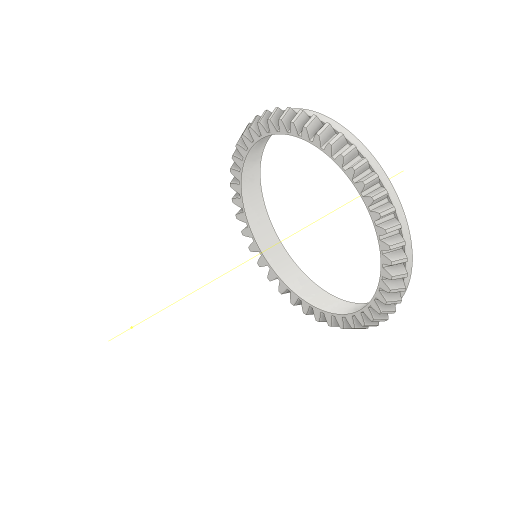
# Autodesk Inventor part: Bevel Gear1
Saved by Autodesk Inventor 2023 (Build 270158000, 158)
## iProperties
CustomPartVersion: 1
Created: 2023-05-08
Part Number: Bevel Gear1
Material: Steel, Mild
Document SubType Name: Modeling
Designer: Juyoung Han
Categories: <?xml version="1.0" encoding="UTF-16"?> <MemberInstance><Categories><FamilyTemplate><FamilyTemplateParameter ValueType="xs:double" Id="1" ObjectReferenceKey="da_z" ObjectType="kUserParameterObject"/><FamilyTemplateParameter ValueType="xs:double" Id="2" ObjectReferenceKey="da_b" ObjectType="kUserParameterObject"/><FamilyTemplateParameter ValueType="xs:double" Id="3" ObjectReferenceKey="da_beta" ObjectType="kUserParameterObject"/><FamilyTemplateParameter ValueType="xs:double" Id="4" ObjectReferenceKey="da_dae" ObjectType="kUserParameterObject"/><FamilyTemplateParameter ValueType="xs:double" Id="5" ObjectReferenceKey="da_ve" ObjectType="kUserParameterObject"/><FamilyTemplateParameter ValueType="xs:double" Id="6" ObjectReferenceKey="da_omega" ObjectType="kUserParameterObject"/><FamilyTemplateParameter ValueType="xs:string" Id="7" ObjectReferenceKey="EAIAABAAAAAAHwAAAAAAAIAAAAAAAAAA" ObjectType="83914240" SubObjectId="SurfaceGeometry"/></FamilyTemplate><ParamToTemplateMap><ParamToTemplate CategoryParameter="//CategoryParameter[@InternalName='046C89C9-8512-4d59-83FE-43B91F4F132A']" TemplateParameter="1"/><ParamToTemplate CategoryParameter="//CategoryParameter[@InternalName='2552DF32-E462-4b46-AEBF-C6C7768E72AC']" TemplateParameter="2"/><ParamToTemplate CategoryParameter="//CategoryParameter[@InternalName='C9EE641D-15FC-4fae-A226-E94C4372FDD7']" TemplateParameter="3"/><ParamToTemplate><ParamToTemplate CategoryParameter="//CategoryParameter[@InternalName='00B6519A-459B-49c7-AD84-2E56D39A5744']" ConstantValue="0.000000"/></ParamToTemplate><ParamToTemplate><ParamToTemplate CategoryParameter="//CategoryParameter[@InternalName='04B31F0E-C7A6-4894-AA32-9629BEFACF47']" ConstantValue="1.000000"/></ParamToTemplate><ParamToTemplate><ParamToTemplate CategoryParameter="//CategoryParameter[@InternalName='43CBEC2E-7847-49e7-A936-2F7889FCB2D9']" ConstantValue="0.200000"/></ParamToTemplate><ParamToTemplate><ParamToTemplate CategoryParameter="//CategoryParameter[@InternalName='B1EFC894-105D-4ebd-86BF-FA20ED196853']" ConstantValue="0.300000"/></ParamToTemplate><ParamToTemplate><ParamToTemplate CategoryParameter="//CategoryParameter[@InternalName='51175063-3D10-4879-93E8-6246FE8B403D']" ConstantValue="2060000000.000000"/></ParamToTemplate><ParamToTemplate><ParamToTemplate CategoryParameter="//CategoryParameter[@InternalName='A3A52E27-4454-46a9-B0BD-C932399B70AF']" ConstantValue="0.300000"/></ParamToTemplate><ParamToTemplate CategoryParameter="//CategoryParameter[@InternalName='2A200944-5A8C-41ca-B96E-8520D2E510F1']" TemplateParameter="4"/><ParamToTemplate><ParamToTemplate CategoryParameter="//CategoryParameter[@InternalName='1A637F62-92C8-44bc-B81F-10802510B579']" ConstantValue="11.345646"/></ParamToTemplate><ParamToTemplate CategoryParameter="//CategoryParameter[@InternalName='B52DD4BE-6863-48fb-BF58-89EF6F9EC65C']" TemplateParameter="5"/><ParamToTemplate><ParamToTemplate CategoryParameter="//CategoryParameter[@InternalName='3956BFF2-84D2-457d-93C2-9B0613DEBA67']" ConstantValue="12.541217"/></ParamToTemplate><ParamToTemplate CategoryParameter="//CategoryParameter[@InternalName='739CFA02-461B-4bf8-8049-181FCAD8B28F']" TemplateParameter="6"/><ParamToTemplate><ParamToTemplate CategoryParameter="//CategoryParameter[@InternalName='A27E999F-E2CE-4481-8A2A-EBF499C4C3C5']" ConstantValue="0.000000"/></ParamToTemplate><ParamToTemplate><ParamToTemplate CategoryParameter="//CategoryParameter[@InternalName='9E1B4470-B2D3-4ff1-B813-535BB4CDF51A']" ConstantValue="3520000.000000"/></ParamToTemplate><ParamToTemplate><ParamToTemplate CategoryParameter="//CategoryParameter[@InternalName='F8452263-BFF6-458c-9FB1-07C4B99E95CD']" ConstantValue="11400000.000000"/></ParamToTemplate><ParamToTemplate><ParamToTemplate CategoryParameter="//CategoryParameter[@InternalName='3E3BB259-FD49-497f-8171-6EBC954A3479']" ConstantValue="2.000000"/></ParamToTemplate><ParamToTemplate CategoryParameter="//CategoryParameter[@InternalName='27C3BAF2-7550-4e4b-AE2C-0DB134B7D9B7']" TemplateParameter="7"/></ParamToTemplateMap><Category DisplayName="Gear" InternalName="DC85795E-93AB-48d5-8EEE-5A27447B64BD" Mnemonic="Gear"><CategoryParameter DisplayName="z" InternalName="046C89C9-8512-4d59-83FE-43B91F4F132A" Mnemonic="z"/><CategoryParameter DisplayName="b" InternalName="2552DF32-E462-4b46-AEBF-C6C7768E72AC" Mnemonic="b"/><CategoryParameter DisplayName="||b|" InternalName="C9EE641D-15FC-4fae-A226-E94C4372FDD7" Mnemonic="beta"/><CategoryParameter DisplayName="x" InternalName="00B6519A-459B-49c7-AD84-2E56D39A5744" Mnemonic="x"/><CategoryParameter DisplayName="a*" InternalName="04B31F0E-C7A6-4894-AA32-9629BEFACF47" Mnemonic="a"/><CategoryParameter DisplayName="c*" InternalName="43CBEC2E-7847-49e7-A936-2F7889FCB2D9" Mnemonic="c"/><CategoryParameter DisplayName="r|.f|*" InternalName="B1EFC894-105D-4ebd-86BF-FA20ED196853" Mnemonic="rf"/><CategoryParameter DisplayName="E" InternalName="51175063-3D10-4879-93E8-6246FE8B403D" Mnemonic="E"/><CategoryParameter DisplayName="||m|" InternalName="A3A52E27-4454-46a9-B0BD-C932399B70AF" Mnemonic="mi"/><Category DisplayName="BevelGear" InternalName="0C98F69A-0C2B-4791-B2FE-7691BB227E77" Mnemonic="BevelGear"><CategoryParameter DisplayName="d|.ae|" InternalName="2A200944-5A8C-41ca-B96E-8520D2E510F1" Mnemonic="dae"/><CategoryParameter DisplayName="d|.ai|" InternalName="1A637F62-92C8-44bc-B81F-10802510B579" Mnemonic="dai"/><CategoryParameter DisplayName="A|.e|" InternalName="B52DD4BE-6863-48fb-BF58-89EF6F9EC65C" Mnemonic="ve"/><CategoryParameter DisplayName="A|.i|" InternalName="3956BFF2-84D2-457d-93C2-9B0613DEBA67" Mnemonic="vi"/><CategoryParameter DisplayName="||S|" InternalName="739CFA02-461B-4bf8-8049-181FCAD8B28F" Mnemonic="omega"/><CategoryParameter DisplayName="x|.t|" InternalName="A27E999F-E2CE-4481-8A2A-EBF499C4C3C5" Mnemonic="xt"/><CategoryParameter DisplayName="||s||.Flim|" InternalName="9E1B4470-B2D3-4ff1-B813-535BB4CDF51A" Mnemonic="sFlim"/><CategoryParameter DisplayName="||s||.Hlim|" InternalName="F8452263-BFF6-458c-9FB1-07C4B99E95CD" Mnemonic="sHlim"/><CategoryParameter DisplayName="type" InternalName="3E3BB259-FD49-497f-8171-6EBC954A3479" Mnemonic="type"/><CategoryParameter DisplayName="PitchDiameter" InternalName="27C3BAF2-7550-4e4b-AE2C-0DB134B7D9B7" Mnemonic="IDS_PITCHDIAM"/></Category></Category></Categories></MemberInstance>
Mass: 523.27 g
Surface Area: 330.412 cm^2
Volume: 66.6586 cm^3
Density: 7.85 g/cm^3
Appearance: Steel
Author: Juyoung Han
Autodesk Inventor part; units mm, degrees
ref_plane "Mesh Plane2" through (0, 0, 0) normal (0.9969173, 0.0784591, 0) x (0, 0, 1)
sketch "Teeth Body Sketch" plane through (0, 0, 0) normal (1, 0, 0) x (0, 1, 0)
  line L0 (0, 0) -> (66.1399, -164.8988) construction
  line L1 (66.1399, -164.8988) -> (73.2167, -161.8642)
  line L2 (73.2167, -161.8642) -> (0, 0) construction
  line L3 (70, -163.2436) -> (0, 0) construction
  line L4 (51.2451, -127.7634) -> (56.7282, -125.4122)
  line L5 (66.1399, -164.8988) -> (51.2451, -127.7634)
  line L6 (73.2167, -161.8642) -> (56.7282, -125.4122)
  line L7 (0, -189.5529) -> (0, 31.5922) projected
  line L8 (0, -163.2436) -> (73.2167, -163.2436) construction
  dimension "d0" = 140
  dimension "d1" = 132.2798
  dimension "d2" = 146.4335
  dimension "d3" = 40
  dimension "d4" = 161.8642
  constraints: 16 end point, 4 point on line, 3 perpendicular, 2 collinear, 1 horizontal alignment, 1 vertical alignment
  measures "d0" diameter of L3.start L7
  measures "d1" diameter of L0.end L7
  measures "d2" diameter of L1.end L7
  measures "d3" distance between parallel lines of L1 L4
  measures "d4" vertical distance of L1.end L0.start
revolve "Teeth Body" add sketch "Teeth Body Sketch" angle 360 about axis through (0, 0, 0) along (0, 0, 1)
ref_plane "Tooth Plane" through (0, 70, -163.2436) normal (0, -0.3941023, 0.9190666) x (1, 0, 0)
sketch "Start Sketch" plane through (0, 70, -163.2436) normal (0, -0.3941023, 0.9190666) x (1, 0, 0)
  line L0 (0, -93.2145) -> (0, 22.3576) projected
  arc A0 (-1.2885, -5.124) -> (-5.8753, 5.5992) centre (-28.0588, -10.2322) ccw
  arc A1 (5.8753, 5.5992) -> (1.2885, -5.124) centre (28.0588, -10.2322) ccw
  line L1 (-1.2885, -5.124) -> (1.2885, -5.124)
  arc A2 (5.8753, 5.5992) -> (-5.8753, 5.5992) centre (0, -76.1642) ccw
  dimension "d7" = 27.2533
  dimension "d8" = 28.0588
  dimension "d9" = 65.932
  dimension "d57" = 81.9742
  dimension "d58" = 71.0402
  constraints: 6 point on circle, 3 centre point, 3 symmetric about line, 2 end point, 1 coincident, 1 perpendicular, 1 other
  measures "d7" radius of A0
  measures "d8" horizontal distance of point (0, -76.164) A0.centre
  measures "d9" vertical distance of point (0, -76.164) A0.centre
  measures "d57" radius of A2
  measures "d58" distance from line of A2.centre L1
sketch "End Sketch" plane through (0, 54.0842, -126.1271) normal (0, -0.3941023, 0.9190666) x (1, 0, 0)
  line L0 (0, -71.2267) -> (0, 17.0838) projected
  arc A0 (-0.9956, -3.959) -> (-4.5394, 4.3261) centre (-21.6791, -7.9057) ccw
  arc A1 (4.5394, 4.3261) -> (0.9956, -3.959) centre (21.6791, -7.9057) ccw
  line L1 (-0.9956, -3.959) -> (0.9956, -3.959)
  arc A2 (4.5394, 4.3261) -> (-4.5394, 4.3261) centre (0, -58.8469) ccw
  dimension "d12" = 21.0567
  dimension "d15" = 21.6791
  dimension "d16" = 50.9411
  dimension "d59" = 63.3358
  dimension "d60" = 54.8879
  constraints: 6 point on circle, 3 centre point, 3 symmetric about line, 2 end point, 1 coincident, 1 other
  measures "d12" radius of A0
  measures "d15" horizontal distance of A0.centre point (0, -58.847)
  measures "d16" vertical distance of A0.centre point (0, -58.847)
  measures "d59" radius of A2
  measures "d60" distance from line of A2.centre L1
loft "Loft" cut profiles "Start Sketch", "End Sketch"
pattern_circular "Circular Pattern" count 40 over 360 about axis through (0, 0, 0) along (0, 0, 1) of "Loft"
ref_plane "End Plane" through (0, 54.0842, -126.1271) normal (0, -0.3941023, 0.9190666) x (1, 0, 0)
sketch3d "3D Sketch Right"
ref_plane "End Plane Right" through (-12.8268, 52.5411, -126.1271) normal (0.0934666, -0.3828585, 0.9190666) x (0.9714698, 0.2371632, 0)
sketch "End Sketch Right" plane through (-12.8268, 52.5411, -126.1271) normal (0.0934666, -0.3828585, 0.9190666) x (0.9714698, 0.2371632, 0)
  arc A0 (-0.9956, -3.959) -> (-4.5394, 4.3261) centre (-21.6791, -7.9057) ccw
  line L0 (0, -84.3011) -> (0, 29.9223) projected
  arc A1 (4.5394, 4.3261) -> (0.9956, -3.959) centre (21.6791, -7.9057) ccw
  line L1 (-0.9956, -3.959) -> (0.9956, -3.959)
  arc A2 (4.5394, 4.3261) -> (-4.5394, 4.3261) centre (0, -58.8469) ccw
  dimension "d70" = 21.6791
  dimension "d71" = 50.9411
  dimension "d72" = 21.0567
  dimension "d73" = 54.8879
  dimension "d74" = 63.3358
  constraints: 6 point on circle, 3 centre point, 3 symmetric about line, 2 end point, 1 coincident, 1 perpendicular, 1 other
  measures "d70" horizontal distance of A2.centre A0.centre
  measures "d71" vertical distance of point (0, -58.847) A0.centre
  measures "d72" radius of A0
  measures "d73" distance from line of point (0, -58.847) L1
  measures "d74" radius of A2
feature "Loft Right" [suppressed]
pattern_circular "Circular Pattern Right" [suppressed]
sketch3d "3D Sketch Left"
ref_plane "End Plane Left" through (12.7774, 52.5411, -126.11) normal (-0.0931208, -0.382915, 0.9190782) x (0.9716797, -0.236302, 0)
sketch "End Sketch Left" plane through (12.7774, 52.5411, -126.11) normal (-0.0931208, -0.382915, 0.9190782) x (0.9716797, -0.236302, 0)
  line L0 (0, -153.675) -> (0, 58.45) projected
  arc A0 (-0.9956, -3.9549) -> (-4.5394, 4.3301) centre (-21.6791, -7.9017) ccw
  arc A1 (4.5394, 4.3301) -> (0.9956, -3.9549) centre (21.6791, -7.9017) ccw
  line L1 (-0.9956, -3.9549) -> (0.9956, -3.9549)
  ellipse E0 centre (0, -49.4218) end of major axis (56.7282, -49.4218) minor radius 52.1377 projected
  arc A2 (4.5394, 4.3301) -> (-4.5394, 4.3301) centre (0, -58.8428) ccw
  dimension "d56" = 52.1377
  dimension "d30" = 21.0567
  dimension "d31" = 21.6791
  dimension "d32" = 50.9411
  dimension "d61" = 63.3358
  dimension "d62" = 54.8879
  constraints: 6 point on circle, 3 centre point, 3 symmetric about line, 2 end point, 1 coincident, 2 other
  measures "d30" radius of A0
  measures "d31" horizontal distance of point (0, -58.843) A0.centre
  measures "d32" vertical distance of A0.centre point (0, -58.843)
  measures "d61" radius of A2
  measures "d62" distance from line of point (0, -58.843) L1
feature "Loft Left" [suppressed]
pattern_circular "Circular Pattern Left" [suppressed]
sketch "Body Sketch" plane through (0, 0, 0) normal (1, 0, 0) x (0, 1, 0)
  line L0 (0, -165.3418) -> (0, -113.6747) projected
  line L1 (66.1399, -164.8988) -> (51.2451, -127.7634) projected
  line L2 (51.2451, -127.7634) -> (0, -127.7634)
  line L3 (66.1399, -164.8988) -> (0, -164.8988)
  constraints: 4 end point, 2 perpendicular, 2 point on line
revolve "Fix Body" add sketch "Body Sketch" angle 360 about axis through (0, 0, 0) along (0, 0, 1)
sketch "Sketch6" plane through (0, 0, 0) normal (1, 0, 0) x (0, 1, 0)
  line L0 (70, -163.2436) -> (0, 0) projected
  line L1 (0, -187.4923) -> (0, 31.2487) projected
surface revolve "Pitch Diameter" sketch "Sketch6" angle 360 about axis through (0, 0, 0) along (0, 0, 1) shown no curves L0
sketch "Sketch8" plane through (0, 0, -127.7634) normal (0, 0, 1) x (0.9969173, 0.0784591, 0)
  circle A0 centre (0, 0) radius 78.8545
  constraints: 1 centre point, 1 coincident
extrude "Extrusion1" cut sketch "Sketch8" along normal blind 10 and the other way blind 25
sketch "Sketch9" plane through (0, 0, -164.8988) normal (0, 0, -1) x (-0.9969173, 0.0784591, 0)
  circle A0 centre (0, 0) radius 68.2
  dimension "d98" = 136.4
  constraints: 1 centre point, 1 coincident
  measures "d98" diameter of A0
extrude "Extrusion2" add sketch "Sketch9" along normal blind 6
sketch "Sketch10" plane through (0, 0, -170.8988) normal (0, 0, -1) x (-1, 0, 0)
  circle A0 centre (0, 0) radius 65.8
  dimension "d101" = 131.6
  constraints: 1 centre point, 1 coincident
  measures "d101" diameter of A0
extrude "Extrusion3" cut sketch "Sketch10" against normal blind 2
sketch "Sketch11" plane through (0, 0, -168.8988) normal (0, 0, -1) x (-1, 0, 0)
  circle A0 centre (0, 0) radius 59.5
  dimension "d104" = 119
  constraints: 1 centre point, 1 coincident
  measures "d104" diameter of A0
extrude "Extrusion4" cut sketch "Sketch11" against normal through all
equation "\"d0\" = da_de"
equation "\"d1\" = da_dfe"
equation "\"d2\" = da_dae"
equation "\"d3\" = da_b"
equation "\"d4\" = da_ve"
equation "\"d7\" = fd_rr"
equation "\"d8\" = fd_x"
equation "\"d9\" = fd_y"
equation "\"d57\" = 0.5 * fd_dva + 0.3 * da_he"
equation "\"d58\" = 0.5 * fd_dva - 1.12 * da_he"
equation "\"da_teethtype\" = 0"
equation "\"da_b\" = 40"
equation "\"da_de\" = 140"
equation "\"da_dae\" = 146.43347"
equation "\"da_dfe\" = 132.27984"
equation "\"da_le\" = 177.61886"
equation "\"da_omega\" = 30deg"
equation "\"da_beta\" = 0"
equation "\"da_delta\" = 23.209998deg"
equation "\"da_alpha\" = 20deg"
equation "\"da_he\" = 7.7"
equation "\"da_ve\" = 161.8642"
equation "\"da_zv\" = 43.522418"
equation "\"fd_loft\" = da_b + 0.05 * da_he"
equation "\"fd_x\" = fd_x1 + fd_x2"
equation "\"fd_y\" = fd_y1 - fd_y2"
equation "\"fd_dd\" = fd_dva - 0.8 * da_he"
equation "\"da_dvw\" = 152.32846"
equation "\"d11\" = fd_loft"
equation "\"da_dm\" = 124.23591"
equation "\"da_x\" = 0"
equation "\"da_m\" = 3.5"
equation "\"d50\" = da_omega"
equation "\"fd_rr\" = 27.253281"
equation "\"fd_dva\" = 159.328463"
equation "\"fd_x1\" = 2.77882"
equation "\"fd_x2\" = 25.280003"
equation "\"fd_y1\" = 76.113523"
equation "\"fd_y2\" = 10.18149"
body "Solid1"
body "Srf1"
